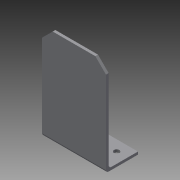
# Autodesk Inventor part: stopper plate
Saved by Autodesk Inventor 2015 SP1 (Build 190203100, 203)
## iProperties
Created: 2015-01-31
Part Number: stopper plate
Material: Generic
Document SubType Name: Modeling
Designer: Admin
Density: 1 g/cm^3
Appearance: Default
Author: Admin
Autodesk Inventor part; units mm, degrees
ref_plane "YZ Plane" through (0, 0, 0) normal (1, 0, 0) x (0, 1, 0)
ref_plane "XZ Plane" through (0, 0, 0) normal (0, 1, 0) x (-1, 0, 0)
ref_plane "XY Plane" through (0, 0, 0) normal (0, 0, 1) x (1, 0, 0)
sketch "Sketch1" plane through (0, 0, 0) normal (1, 0, 0) x (0, 1, 0)
  line L0 (0, 0) -> (114.3, 0)
  line L1 (114.3, 0) -> (114.3, -3.175)
  line L2 (114.3, -3.175) -> (0, -3.175)
  line L3 (0, -3.175) -> (0, 0)
  line L4 (0, 0) -> (3.175, 0)
  line L5 (3.175, 0) -> (3.175, -31.75)
  line L6 (3.175, -31.75) -> (0, -31.75)
  line L7 (0, -31.75) -> (0, 0)
  dimension "d0" = 114.3
  dimension "d1" = 3.175
  dimension "d2" = 3.175
  dimension "d3" = 31.75
  constraints: 16 end point, 4 parallel, 2 horizontal, 2 perpendicular
  measures "d0" distance of L1.end L2.end
  measures "d1" distance of L0.end L1.end
  measures "d2" distance of L5.end L6.end
  measures "d3" distance of L4.end L5.end
extrude "Extrusion1" add sketch "Sketch1" along normal blind 76.2
sketch "Sketch2" plane through (0, 0, -31.75) normal (0, -1, 0) x (1, 0, 0)
  line L0 (76.2, 31.75) -> (76.2, 0) projected
  line L1 (0, 31.75) -> (0, 0) projected
  line L2 (0, 0) -> (76.2, 0) projected
  point P0 (63.5, 12.7)
  point P1 (12.7, 12.7)
  dimension "d6" = 12.7
  dimension "d7" = 12.7
  dimension "d8" = 12.7
  dimension "d9" = 12.7
  measures "d6" distance from line of L2 point (63.5, 12.7)
  measures "d7" distance from line of L0 point (63.5, 12.7)
  measures "d8" distance from line of L1 point (12.7, 12.7)
  measures "d9" distance from line of L2 point (12.7, 12.7)
hole "Hole1" at (63.5, 0, -19.05) at (12.7, 0, -19.05) direction (0, 1, 0) diameter 6.35 end through all
fillet "Fillet1" radius 3.175 2 edges at (38.1, 0, 0) (38.1, 3.175, -3.175)
chamfer "Chamfer1" distance 12.7 angle 45 2 edges at (76.2, 114.3, -1.5875) (0, 114.3, -1.5875)
body "Solid1"
